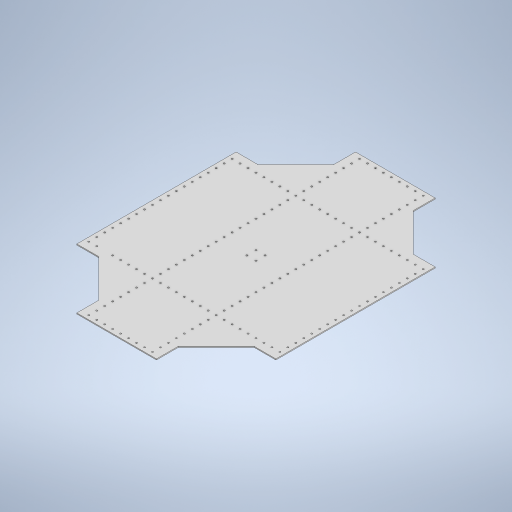
# Autodesk Inventor part: Baseplate V2.1
Saved by Autodesk Inventor 2023.2 (Build 272271000, 271)
## iProperties
Created: 2023-01-16
Part Number: Baseplate V2.1
Material: Generic
Document SubType Name: Modeling
Designer: Gabriel - T3 CAD
Density: 1 g/cm^3
Appearance: Default
Author: Gabriel - T3 CAD
Autodesk Inventor part; units mm, degrees
ref_plane "YZ Plane" through (0, 0, 0) normal (1, 0, 0) x (0, 1, 0)
ref_plane "XZ Plane" through (0, 0, 0) normal (0, 1, 0) x (-1, 0, 0)
ref_plane "XY Plane" through (0, 0, 0) normal (0, 0, 1) x (1, 0, 0)
sketch "Sketch1" plane through (0, 0, 0) normal (0, 1, 0) x (-1, 0, 0)
  line L0 (0, 0) -> (635, 0)
  line L1 (635, 0) -> (635, 889)
  line L2 (635, 889) -> (0, 889)
  line L3 (0, 889) -> (0, 0)
  line L4 (0, 0) -> (69.85, 0)
  line L5 (69.85, 0) -> (69.85, 190.5)
  line L6 (69.85, 190.5) -> (0, 190.5)
  line L7 (0, 190.5) -> (0, 0)
  line L8 (0, 0) -> (190.5, 0)
  line L9 (190.5, 0) -> (190.5, 69.85)
  line L10 (190.5, 69.85) -> (0, 69.85)
  line L11 (0, 69.85) -> (0, 0)
  line L12 (190.5, 69.85) -> (69.85, 190.5)
  line L13 (317.5, 889) -> (317.5, 0)
  line L14 (0, 444.5) -> (635, 444.5)
  line L15 (565.15, 0) -> (565.15, 190.5)
  line L16 (565.15, 190.5) -> (635, 190.5)
  line L17 (444.5, 0) -> (444.5, 69.85)
  line L18 (444.5, 69.85) -> (635, 69.85)
  line L19 (444.5, 69.85) -> (565.15, 190.5)
  line L20 (69.85, 889) -> (69.85, 698.5)
  line L21 (69.85, 698.5) -> (0, 698.5)
  line L22 (190.5, 889) -> (190.5, 819.15)
  line L23 (190.5, 819.15) -> (0, 819.15)
  line L24 (190.5, 819.15) -> (69.85, 698.5)
  line L25 (565.15, 889) -> (565.15, 698.5)
  line L26 (565.15, 698.5) -> (635, 698.5)
  line L27 (444.5, 889) -> (444.5, 819.15)
  line L28 (444.5, 819.15) -> (635, 819.15)
  line L29 (444.5, 819.15) -> (565.15, 698.5)
  circle A0 centre (622.3, 876.3) radius 2.5797
  circle A1 centre (622.3, 850.9) radius 2.5797
  circle A2 centre (622.3, 825.5) radius 2.5797
  circle A3 centre (622.3, 800.1) radius 2.5797
  circle A4 centre (622.3, 774.7) radius 2.5797
  circle A5 centre (622.3, 749.3) radius 2.5797
  circle A6 centre (622.3, 723.9) radius 2.5797
  circle A7 centre (622.3, 698.5) radius 2.5797
  circle A8 centre (622.3, 673.1) radius 2.5797
  circle A9 centre (622.3, 647.7) radius 2.5797
  circle A10 centre (622.3, 622.3) radius 2.5797
  circle A11 centre (622.3, 596.9) radius 2.5797
  circle A12 centre (622.3, 571.5) radius 2.5797
  circle A13 centre (622.3, 546.1) radius 2.5797
  circle A14 centre (622.3, 520.7) radius 2.5797
  circle A15 centre (622.3, 495.3) radius 2.5797
  circle A16 centre (622.3, 469.9) radius 2.5797
  circle A17 centre (622.3, 444.5) radius 2.5797
  circle A18 centre (622.3, 419.1) radius 2.5797
  circle A19 centre (622.3, 393.7) radius 2.5797
  circle A20 centre (622.3, 368.3) radius 2.5797
  circle A21 centre (622.3, 342.9) radius 2.5797
  circle A22 centre (622.3, 317.5) radius 2.5797
  circle A23 centre (622.3, 292.1) radius 2.5797
  circle A24 centre (622.3, 266.7) radius 2.5797
  circle A25 centre (622.3, 241.3) radius 2.5797
  circle A26 centre (622.3, 215.9) radius 2.5797
  circle A27 centre (622.3, 190.5) radius 2.5797
  circle A28 centre (622.3, 165.1) radius 2.5797
  circle A29 centre (622.3, 139.7) radius 2.5797
  circle A30 centre (622.3, 114.3) radius 2.5797
  circle A31 centre (622.3, 88.9) radius 2.5797
  circle A32 centre (622.3, 63.5) radius 2.5797
  circle A33 centre (622.3, 38.1) radius 2.5797
  circle A34 centre (622.3, 12.7) radius 2.5797
  circle A35 centre (12.7, 876.3) radius 2.5797
  circle A36 centre (12.7, 850.9) radius 2.5797
  circle A37 centre (12.7, 825.5) radius 2.5797
  circle A38 centre (12.7, 800.1) radius 2.5797
  circle A39 centre (12.7, 774.7) radius 2.5797
  circle A40 centre (12.7, 749.3) radius 2.5797
  circle A41 centre (12.7, 723.9) radius 2.5797
  circle A42 centre (12.7, 698.5) radius 2.5797
  circle A43 centre (12.7, 673.1) radius 2.5797
  circle A44 centre (12.7, 647.7) radius 2.5797
  circle A45 centre (12.7, 622.3) radius 2.5797
  circle A46 centre (12.7, 596.9) radius 2.5797
  circle A47 centre (12.7, 571.5) radius 2.5797
  circle A48 centre (12.7, 546.1) radius 2.5797
  circle A49 centre (12.7, 520.7) radius 2.5797
  circle A50 centre (12.7, 495.3) radius 2.5797
  circle A51 centre (12.7, 469.9) radius 2.5797
  circle A52 centre (12.7, 444.5) radius 2.5797
  circle A53 centre (12.7, 419.1) radius 2.5797
  circle A54 centre (12.7, 393.7) radius 2.5797
  circle A55 centre (12.7, 368.3) radius 2.5797
  circle A56 centre (12.7, 342.9) radius 2.5797
  circle A57 centre (12.7, 317.5) radius 2.5797
  circle A58 centre (12.7, 292.1) radius 2.5797
  circle A59 centre (12.7, 266.7) radius 2.5797
  circle A60 centre (12.7, 241.3) radius 2.5797
  circle A61 centre (12.7, 215.9) radius 2.5797
  circle A62 centre (12.7, 190.5) radius 2.5797
  circle A63 centre (12.7, 165.1) radius 2.5797
  circle A64 centre (12.7, 139.7) radius 2.5797
  circle A65 centre (12.7, 114.3) radius 2.5797
  circle A66 centre (12.7, 88.9) radius 2.5797
  circle A67 centre (12.7, 63.5) radius 2.5797
  circle A68 centre (12.7, 38.1) radius 2.5797
  circle A69 centre (12.7, 12.7) radius 2.5797
  circle A70 centre (596.9, 876.3) radius 2.5797
  circle A71 centre (571.5, 876.3) radius 2.5797
  circle A72 centre (546.1, 876.3) radius 2.5797
  circle A73 centre (520.7, 876.3) radius 2.5797
  circle A74 centre (495.3, 876.3) radius 2.5797
  circle A75 centre (469.9, 876.3) radius 2.5797
  circle A76 centre (444.5, 876.3) radius 2.5797
  circle A77 centre (419.1, 876.3) radius 2.5797
  circle A78 centre (393.7, 876.3) radius 2.5797
  circle A79 centre (368.3, 876.3) radius 2.5797
  circle A80 centre (342.9, 876.3) radius 2.5797
  circle A81 centre (317.5, 876.3) radius 2.5797
  circle A82 centre (292.1, 876.3) radius 2.5797
  circle A83 centre (266.7, 876.3) radius 2.5797
  circle A84 centre (241.3, 876.3) radius 2.5797
  circle A85 centre (215.9, 876.3) radius 2.5797
  circle A86 centre (190.5, 876.3) radius 2.5797
  circle A87 centre (165.1, 876.3) radius 2.5797
  circle A88 centre (139.7, 876.3) radius 2.5797
  circle A89 centre (114.3, 876.3) radius 2.5797
  circle A90 centre (88.9, 876.3) radius 2.5797
  circle A91 centre (63.5, 876.3) radius 2.5797
  circle A92 centre (38.1, 876.3) radius 2.5797
  circle A93 centre (12.7, 876.3) radius 2.5797
  circle A94 centre (622.3, 12.7) radius 2.5797
  circle A95 centre (596.9, 12.7) radius 2.5797
  circle A96 centre (571.5, 12.7) radius 2.5797
  circle A97 centre (546.1, 12.7) radius 2.5797
  circle A98 centre (520.7, 12.7) radius 2.5797
  circle A99 centre (495.3, 12.7) radius 2.5797
  circle A100 centre (469.9, 12.7) radius 2.5797
  circle A101 centre (444.5, 12.7) radius 2.5797
  circle A102 centre (419.1, 12.7) radius 2.5797
  circle A103 centre (393.7, 12.7) radius 2.5797
  circle A104 centre (368.3, 12.7) radius 2.5797
  circle A105 centre (342.9, 12.7) radius 2.5797
  circle A106 centre (317.5, 12.7) radius 2.5797
  circle A107 centre (292.1, 12.7) radius 2.5797
  circle A108 centre (266.7, 12.7) radius 2.5797
  circle A109 centre (241.3, 12.7) radius 2.5797
  circle A110 centre (215.9, 12.7) radius 2.5797
  circle A111 centre (190.5, 12.7) radius 2.5797
  circle A112 centre (165.1, 12.7) radius 2.5797
  circle A113 centre (139.7, 12.7) radius 2.5797
  circle A114 centre (114.3, 12.7) radius 2.5797
  circle A115 centre (88.9, 12.7) radius 2.5797
  circle A116 centre (63.5, 12.7) radius 2.5797
  circle A117 centre (38.1, 12.7) radius 2.5797
  circle A118 centre (12.7, 12.7) radius 2.5797
  point P0 (0, 698.5)
  dimension "d0" = 635
  dimension "d1" = 889
  dimension "d2" = 69.85
  dimension "d3" = 190.5
  dimension "d4" = 190.5
  dimension "d5" = 69.85
  dimension "d6" = 317.5
  dimension "d7" = 444.5
  dimension "d8" = 12.7
  dimension "d9" = 12.7
  dimension "d10" = 5.1594
  dimension "d13" = 25.4
  dimension "d16" = 609.6
  dimension "d21" = 25.4
  dimension "d24" = 863.6
  constraints: 119 centre point, 60 end point, 18 symmetric about line, 6 parallel, 5 horizontal, 5 perpendicular, 4 midpoint, 2 vertical, 236 other
  measures "d0" distance of L2.end L1.end
  measures "d1" distance of L1.end L0.end
  measures "d2" distance of L6.end L5.end
  measures "d3" distance of L5.end L4.end
  measures "d4" distance of L10.end L9.end
  measures "d5" distance of L9.end L8.end
  measures "d6" distance between parallel lines of L3 L13
  measures "d7" distance between parallel lines of L2 L14
  measures "d8" distance from line of A0.centre L1
  measures "d9" distance from line of L2 A0.centre
  measures "d10" diameter of A0
  measures "d13" distance of A0.centre A1.centre
  measures "d16" distance of A0.centre A35.centre
  measures "d21" distance of A0.centre A70.centre
  measures "d24" distance of A0.centre A94.centre
extrude "Extrusion1" add sketch "Sketch1" along normal blind 3.175 contours L9 A111 L12 L6 A62 L3 L14 A52 L13 A106 L0 | L13 A106 L14 A17 L1 L16 A27 L19 L17 A101 L0 | L9 A111 | L3 L21 A42 L24 L22 A86 L2 L13 A81 L14 A52 | A62 L6 | A101 L17 | L21 A42 | L13 A81 L2 L27 A76 L29 L26 A7 L1 L14 A17 | A27 L16 | L22 A86 | A7 L26 | L27 A76 picked at (191.3383, 12.5087) picked at (13.5349, 190.7058) picked at (444.2942, 11.8651) picked at (12.8036, 697.6464) picked at (622.9436, 191.4818) picked at (191.721, 876.4913) picked at (621.9951, 697.696) picked at (443.5182, 875.6564)
sketch "Sketch4" plane through (0, 3.175, 0) normal (0, 1, 0) x (1, 0, 0)
  line L0 (-331.978, -458.978) -> (-303.022, -458.978)
  line L1 (-303.022, -458.978) -> (-303.022, -430.022)
  line L2 (-303.022, -430.022) -> (-331.978, -430.022)
  line L3 (-331.978, -430.022) -> (-331.978, -458.978)
  circle A0 centre (-303.022, -430.022) radius 2.5797
  circle A1 centre (-331.978, -430.022) radius 2.5797
  circle A2 centre (-331.978, -458.978) radius 2.5797
  circle A3 centre (-303.022, -458.978) radius 2.5797
  line L4 (0, -698.5) -> (0, -190.5) projected
  line L5 (-190.5, 0) -> (-444.5, 0) projected
  point P0 (0, 0)
  dimension "d53" = 28.956
  dimension "d54" = 28.956
  dimension "d55" = 5.1594
  dimension "d56" = 5.1594
  dimension "d57" = 5.1594
  dimension "d58" = 5.1594
  dimension "d59" = 303.022
  dimension "d60" = 430.022
  constraints: 8 end point, 4 centre point, 4 coincident, 2 parallel, 1 horizontal, 1 perpendicular
  measures "d53" distance of L1.end L2.end
  measures "d54" distance of L0.end L1.end
  measures "d55" diameter of A3
  measures "d56" diameter of A2
  measures "d57" diameter of A1
  measures "d58" diameter of A0
  measures "d59" distance between parallel lines of L4 L1
  measures "d60" distance between parallel lines of L5 L2
extrude "Extrusion4" cut sketch "Sketch4" against normal blind 25.4 contours L3 A2 L0 | L0 A2 L3 | A3 L1 L0 | L0 L1 A3 | A1 L2 L3 | L3 L2 A1 | A0 L2 L1 | L1 L2 A0
sketch "Sketch5" plane through (0, 3.175, 0) normal (0, 1, 0) x (1, 0, 0)
  circle A0 centre (-215.9, -12.7) radius 2.5797
  line L0 (-190.5, -69.85) -> (-190.5, 0) projected
  line L1 (-190.5, 0) -> (-444.5, 0) projected
  circle A1 centre (-215.9, -38.1) radius 2.5797
  circle A2 centre (-215.9, -63.5) radius 2.5797
  circle A3 centre (-215.9, -88.9) radius 2.5797
  circle A4 centre (-215.9, -114.3) radius 2.5797
  circle A5 centre (-215.9, -139.7) radius 2.5797
  circle A6 centre (-215.9, -165.1) radius 2.5797
  circle A7 centre (-215.9, -190.5) radius 2.5797
  circle A8 centre (-215.9, -215.9) radius 2.5797
  circle A9 centre (-215.9, -241.3) radius 2.5797
  circle A10 centre (-215.9, -266.7) radius 2.5797
  circle A11 centre (-215.9, -292.1) radius 2.5797
  circle A12 centre (-215.9, -317.5) radius 2.5797
  circle A13 centre (-215.9, -342.9) radius 2.5797
  circle A14 centre (-215.9, -368.3) radius 2.5797
  circle A15 centre (-215.9, -393.7) radius 2.5797
  circle A16 centre (-215.9, -419.1) radius 2.5797
  circle A17 centre (-215.9, -444.5) radius 2.5797
  circle A18 centre (-215.9, -469.9) radius 2.5797
  circle A19 centre (-215.9, -495.3) radius 2.5797
  circle A20 centre (-215.9, -520.7) radius 2.5797
  circle A21 centre (-215.9, -546.1) radius 2.5797
  circle A22 centre (-215.9, -571.5) radius 2.5797
  circle A23 centre (-215.9, -596.9) radius 2.5797
  circle A24 centre (-215.9, -622.3) radius 2.5797
  circle A25 centre (-215.9, -647.7) radius 2.5797
  circle A26 centre (-215.9, -673.1) radius 2.5797
  circle A27 centre (-215.9, -698.5) radius 2.5797
  circle A28 centre (-215.9, -723.9) radius 2.5797
  circle A29 centre (-215.9, -749.3) radius 2.5797
  circle A30 centre (-215.9, -774.7) radius 2.5797
  circle A31 centre (-215.9, -800.1) radius 2.5797
  circle A32 centre (-215.9, -825.5) radius 2.5797
  circle A33 centre (-215.9, -850.9) radius 2.5797
  circle A34 centre (-215.9, -876.3) radius 2.5797
  circle A35 centre (-419.1, -12.7) radius 2.5797
  circle A36 centre (-419.1, -38.1) radius 2.5797
  circle A37 centre (-419.1, -63.5) radius 2.5797
  circle A38 centre (-419.1, -88.9) radius 2.5797
  circle A39 centre (-419.1, -114.3) radius 2.5797
  circle A40 centre (-419.1, -139.7) radius 2.5797
  circle A41 centre (-419.1, -165.1) radius 2.5797
  circle A42 centre (-419.1, -190.5) radius 2.5797
  circle A43 centre (-419.1, -215.9) radius 2.5797
  circle A44 centre (-419.1, -241.3) radius 2.5797
  circle A45 centre (-419.1, -266.7) radius 2.5797
  circle A46 centre (-419.1, -292.1) radius 2.5797
  circle A47 centre (-419.1, -317.5) radius 2.5797
  circle A48 centre (-419.1, -342.9) radius 2.5797
  circle A49 centre (-419.1, -368.3) radius 2.5797
  circle A50 centre (-419.1, -393.7) radius 2.5797
  circle A51 centre (-419.1, -419.1) radius 2.5797
  circle A52 centre (-419.1, -444.5) radius 2.5797
  circle A53 centre (-419.1, -469.9) radius 2.5797
  circle A54 centre (-419.1, -495.3) radius 2.5797
  circle A55 centre (-419.1, -520.7) radius 2.5797
  circle A56 centre (-419.1, -546.1) radius 2.5797
  circle A57 centre (-419.1, -571.5) radius 2.5797
  circle A58 centre (-419.1, -596.9) radius 2.5797
  circle A59 centre (-419.1, -622.3) radius 2.5797
  circle A60 centre (-419.1, -647.7) radius 2.5797
  circle A61 centre (-419.1, -673.1) radius 2.5797
  circle A62 centre (-419.1, -698.5) radius 2.5797
  circle A63 centre (-419.1, -723.9) radius 2.5797
  circle A64 centre (-419.1, -749.3) radius 2.5797
  circle A65 centre (-419.1, -774.7) radius 2.5797
  circle A66 centre (-419.1, -800.1) radius 2.5797
  circle A67 centre (-419.1, -825.5) radius 2.5797
  circle A68 centre (-419.1, -850.9) radius 2.5797
  circle A69 centre (-419.1, -876.3) radius 2.5797
  circle A70 centre (-12.7, -215.9) radius 2.5797
  line L2 (0, -698.5) -> (0, -190.5) projected
  circle A71 centre (-12.7, -673.1) radius 2.5797
  circle A72 centre (-38.1, -215.9) radius 2.5797
  circle A73 centre (-38.1, -673.1) radius 2.5797
  circle A74 centre (-63.5, -215.9) radius 2.5797
  circle A75 centre (-63.5, -673.1) radius 2.5797
  circle A76 centre (-88.9, -215.9) radius 2.5797
  circle A77 centre (-88.9, -673.1) radius 2.5797
  circle A78 centre (-114.3, -215.9) radius 2.5797
  circle A79 centre (-114.3, -673.1) radius 2.5797
  circle A80 centre (-139.7, -215.9) radius 2.5797
  circle A81 centre (-139.7, -673.1) radius 2.5797
  circle A82 centre (-165.1, -215.9) radius 2.5797
  circle A83 centre (-165.1, -673.1) radius 2.5797
  circle A84 centre (-190.5, -215.9) radius 2.5797
  circle A85 centre (-190.5, -673.1) radius 2.5797
  circle A86 centre (-215.9, -215.9) radius 2.5797
  circle A87 centre (-215.9, -673.1) radius 2.5797
  circle A88 centre (-241.3, -215.9) radius 2.5797
  circle A89 centre (-241.3, -673.1) radius 2.5797
  circle A90 centre (-266.7, -215.9) radius 2.5797
  circle A91 centre (-266.7, -673.1) radius 2.5797
  circle A92 centre (-292.1, -215.9) radius 2.5797
  circle A93 centre (-292.1, -673.1) radius 2.5797
  circle A94 centre (-317.5, -215.9) radius 2.5797
  circle A95 centre (-317.5, -673.1) radius 2.5797
  circle A96 centre (-342.9, -215.9) radius 2.5797
  circle A97 centre (-342.9, -673.1) radius 2.5797
  circle A98 centre (-368.3, -215.9) radius 2.5797
  circle A99 centre (-368.3, -673.1) radius 2.5797
  circle A100 centre (-393.7, -215.9) radius 2.5797
  circle A101 centre (-393.7, -673.1) radius 2.5797
  circle A102 centre (-419.1, -215.9) radius 2.5797
  circle A103 centre (-419.1, -673.1) radius 2.5797
  circle A104 centre (-444.5, -215.9) radius 2.5797
  circle A105 centre (-444.5, -673.1) radius 2.5797
  circle A106 centre (-469.9, -215.9) radius 2.5797
  circle A107 centre (-469.9, -673.1) radius 2.5797
  circle A108 centre (-495.3, -215.9) radius 2.5797
  circle A109 centre (-495.3, -673.1) radius 2.5797
  circle A110 centre (-520.7, -215.9) radius 2.5797
  circle A111 centre (-520.7, -673.1) radius 2.5797
  circle A112 centre (-546.1, -215.9) radius 2.5797
  circle A113 centre (-546.1, -673.1) radius 2.5797
  circle A114 centre (-571.5, -215.9) radius 2.5797
  circle A115 centre (-571.5, -673.1) radius 2.5797
  circle A116 centre (-596.9, -215.9) radius 2.5797
  circle A117 centre (-596.9, -673.1) radius 2.5797
  circle A118 centre (-622.3, -215.9) radius 2.5797
  circle A119 centre (-622.3, -673.1) radius 2.5797
  point P0 (0, 0)
  dimension "d63" = 25.4
  dimension "d64" = 12.7
  dimension "d65" = 5.1594
  dimension "d68" = 25.4
  dimension "d71" = 203.2
  dimension "d76" = 215.9
  dimension "d77" = 12.7
  dimension "d78" = 5.1594
  dimension "d81" = 457.2
  dimension "d84" = 25.4
  constraints: 120 centre point, 2 horizontal, 2 vertical, 236 other
  measures "d63" distance from line of A0.centre L0
  measures "d64" distance from line of L1 A0.centre
  measures "d65" diameter of A0
  measures "d68" distance of A0.centre A1.centre
  measures "d71" distance of A0.centre A35.centre
  measures "d76" vertical distance of point (0, 0) A70.centre
  measures "d77" distance from line of L2 A70.centre
  measures "d78" diameter of A70
  measures "d81" distance of A70.centre A71.centre
  measures "d84" distance of A70.centre A72.centre
extrude "Extrusion5" cut sketch "Sketch5" against normal blind 25.4 contours A0 | A1 | A2 | A3 | A4 | A5 | A6 | A7 | A8 | A9 | A10 | A11 | A12 | A13 | A14 | A15 | A16 | A17 | A18 | A19 | A20 | A21 | A22 | A23 | A24 | A25 | A26 | A27 | A28 | A29 | A30 | A31 | A32 | A33 | A34 | A35 | A36 | A37 | A38 | A39 | A40 | A41 | A42 | A43 | A44 | A45 | A46 | A47 | A48 | A49 | A50 | A51 | A52 | A53 | A54 | A55 | A56 | A57 | A58 | A59 | A60 | A61 | A62 | A63 | A64 | A65 | A66 | A67 | A68 | A69 | A70 | A71 | A72 | A73 | A74 | A75 | A76 | A77 | A78 | A79 | A80 | A81 | A82 | A83 | A84 | A85 | A88 | A89 | A90 | A91 | A92 | A93 | A94 | A95 | A96 | A97 | A98 | A99 | A100 | A101 | A104 | A105 | A106 | A107 | A108 | A109 | A110 | A111 | A112 | A113 | A114 | A116 | A117 | A118 | A119
equation "\"d6\" = 0.5 * d0"
equation "\"d7\" = 0.5 * d1"
equation "\"d54\" = d53"
equation "\"d56\" = d55"
equation "\"d57\" = d55"
equation "\"d58\" = d55"
body "Solid1"
